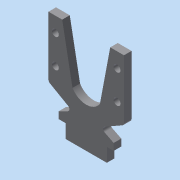
# Autodesk Inventor part: sables
Saved by Autodesk Inventor 2015 (Build 190159000, 159)
## iProperties
Created: 2017-09-29
Part Number: sables
Material: Generic
Document SubType Name: Modeling
Designer: Max
Density: 1 g/cm^3
Appearance: Default
Author: Max
Autodesk Inventor part; units mm, degrees
ref_plane "YZ Plane" through (0, 0, 0) normal (1, 0, 0) x (0, 1, 0)
ref_plane "XZ Plane" through (0, 0, 0) normal (0, 1, 0) x (-1, 0, 0)
ref_plane "XY Plane" through (0, 0, 0) normal (0, 0, 1) x (1, 0, 0)
sketch "Sketch3" plane through (0, 0, 0) normal (0, 0, 1) x (1, 0, 0)
  line L0 (-10, 20) -> (-20, 15)
  line L1 (-10, 20) -> (-27.4665, 29.933)
  line L2 (-27.4665, 29.933) -> (-27.4665, 73.9793)
  line L3 (-27.4665, 73.9793) -> (-17.4665, 73.9793)
  line L4 (-17.4665, 73.9793) -> (-10, 34.7248)
  line L5 (10, 20) -> (20, 15)
  line L6 (10, 20) -> (27.4665, 29.933)
  line L7 (27.4665, 29.933) -> (27.4665, 73.9793)
  line L8 (27.4665, 73.9793) -> (17.4665, 73.9793)
  line L9 (17.4665, 73.9793) -> (10, 34.7248)
  circle A0 centre (-22.4665, 63.181) radius 2.5
  circle A1 centre (-22.4665, 42.2172) radius 2.5
  circle A2 centre (22.4665, 63.181) radius 2.5
  circle A3 centre (22.4665, 42.2172) radius 2.5
  arc A4 (-10, 34.7248) -> (10, 34.7248) centre (0, 40.7878) ccw
  line L10 (-20, 15) -> (-20, 10)
  line L11 (-20, 10) -> (-15, 10)
  line L12 (-15, 10) -> (-15, 0)
  line L13 (-15, 0) -> (15, 0)
  line L14 (15, 0) -> (15, 10)
  line L15 (15, 10) -> (20, 10)
  line L16 (20, 10) -> (20, 15)
  point P0 (0, 0)
  dimension "d2" = 10
  dimension "d3" = 5
  dimension "d4" = 5
  dimension "d9" = 5
  dimension "d10" = 5
  dimension "d11" = 30
  dimension "d12" = 90
  dimension "d13" = 5
  constraints: 34 end point, 6 perpendicular, 5 centre point, 2 point on circle, 2 point on line, 2 vertical
  measures "d2" distance of L2.end L3.end
  measures "d3" diameter of A0
  measures "d4" diameter of A1
  measures "d9" distance of L0.end L10.end
  measures "d10" distance of L10.end L11.end
  measures "d11" distance of L12.end L13.end
  measures "d12" angle of L13 L12
  measures "d13" distance of L14.end L15.end
extrude "Extrusion1" add sketch "Sketch3" along normal blind 5.5
fillet "Fillet1" radius 2 4 edges at (27.4665, 29.933, 2.75) (-27.4665, 29.933, 2.75) (-10, 20, 2.75) (10, 20, 2.75)
body "Solid1"
